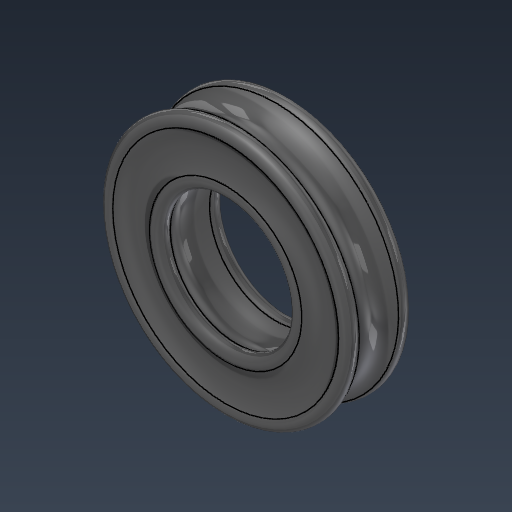
# Autodesk Inventor part: X-Ring 5.94x3.53
Saved by Autodesk Inventor 2023.1 (Build 271208000, 208)
## iProperties
Created: 2015-08-15
Part Number: X-Ring 5.94x3.53
Material: Gummi, Silikon
Document SubType Name: Modeling
Designer: rYan
Mass: 0.334872 g
Surface Area: 4.61579 cm^2
Volume: 0.267898 cm^3
Density: 1.25 g/cm^3
Appearance: Gummi - schwarz - Version 1.1
Author: rYan
Autodesk Inventor part; units mm, degrees
ref_plane "YZ Plane" through (0, 0, 0) normal (1, 0, 0) x (0, 1, 0)
ref_plane "XZ Plane" through (0, 0, 0) normal (0, 1, 0) x (-1, 0, 0)
ref_plane "XY Plane" through (0, 0, 0) normal (0, 0, 1) x (1, 0, 0)
sketch "Skizze1" plane through (0, 0, 0) normal (1, 0, 0) x (0, 1, 0)
  arc A0 (-1.0776, 6.7282) -> (-1.6616, 6.1816) centre (-1.365, 6.45) ccw
  arc A1 (-1.0776, 6.7282) -> (1.0776, 6.7282) centre (0, 7.7717) ccw
  arc A2 (1.6616, 6.1816) -> (1.0776, 6.7282) centre (1.365, 6.45) ccw
  arc A3 (1.6616, 6.1816) -> (1.6616, 4.1684) centre (2.7737, 5.175) ccw
  arc A4 (1.0776, 3.6218) -> (1.6616, 4.1684) centre (1.365, 3.9) ccw
  arc A5 (1.0776, 3.6218) -> (-1.0776, 3.6218) centre (0, 2.5783) ccw
  arc A6 (-1.6616, 4.1684) -> (-1.0776, 3.6218) centre (-1.365, 3.9) ccw
  arc A7 (-1.6616, 4.1684) -> (-1.6616, 6.1816) centre (-2.7737, 5.175) ccw
  line L0 (-1.365, 6.45) -> (1.365, 6.45) construction
  line L1 (1.365, 6.45) -> (1.365, 3.9) construction
  line L2 (1.365, 3.9) -> (-1.365, 3.9) construction
  line L3 (-1.365, 3.9) -> (-1.365, 6.45) construction
  line L4 (0, 9.326) -> (0, -1.5543) projected
  line L5 (-3.8831, 0) -> (3.8831, 0) construction
  line L6 (0, 6.45) -> (0, 3.9) construction
  line L7 (-1.365, 5.175) -> (1.365, 5.175) construction
  line L8 (-1.365, 6.45) -> (-1.765, 6.45) construction
  line L9 (-1.365, 3.9) -> (-1.765, 3.9) construction
  line L10 (-1.765, 3.9) -> (-1.765, 6.45) construction
  line L11 (-1.365, 6.45) -> (-1.365, 6.85) construction
  line L12 (-1.365, 3.9) -> (-1.365, 3.5) construction
  line L13 (1.365, 3.9) -> (1.365, 3.5) construction
  line L14 (-1.365, 3.5) -> (1.365, 3.5) construction
  line L15 (1.365, 6.45) -> (1.765, 6.45) construction
  line L16 (1.365, 3.9) -> (1.765, 3.9) construction
  line L17 (-1.365, 6.85) -> (1.365, 6.85) construction
  point P0 (0, 0)
  dimension "d0" = 3.35
  dimension "d1" = 7
  dimension "d2" = 3.53
  dimension "d3" = 1.5
  dimension "d4" = 0.4
  constraints: 32 end point, 25 point on circle, 10 tangent, 8 centre point, 7 parallel, 4 horizontal, 4 midpoint, 2 equal radius, 2 vertical, 1 point on line, 3 other
  measures "d0" distance of L12.end L11.end
  measures "d1" diameter of L14 L5
  measures "d2" distance of L8.end L15.end
  measures "d3" radius of A7
  measures "d4" radius of A0
revolve "Umdrehung1" add sketch "Skizze1" angle 360 about axis through (0, 0, 0) along (0, 1, 0)
